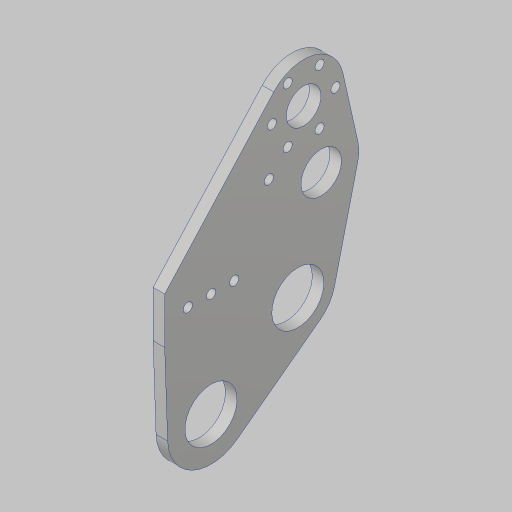
# Autodesk Inventor part: GP5-004
Saved by Autodesk Inventor 2023.5 (Build 275446000, 446)
## iProperties
Created: 2025-02-03
Part Number: GP5-004
Material: Aluminum 6061
Document SubType Name: Modeling
Designer: slick
Density: 2.7 g/cm^3
Appearance: Aluminum - Flat
Author: slick
Autodesk Inventor part; units mm, degrees
ref_plane "YZ Plane" through (0, 0, 0) normal (1, 0, 0) x (0, 1, 0)
ref_plane "XZ Plane" through (0, 0, 0) normal (0, 1, 0) x (-1, 0, 0)
ref_plane "XY Plane" through (0, 0, 0) normal (0, 0, 1) x (1, 0, 0)
sketch "Sketch1" plane through (0, 0, 0) normal (1, 0, 0) x (0, 1, 0)
  line L0 (-12.7, 25.4) -> (12.7, 25.4) construction
  line L1 (12.7, 25.4) -> (12.7, -25.4) construction
  line L2 (12.7, -25.4) -> (-12.7, -25.4) construction
  line L3 (-12.7, -25.4) -> (-12.7, 25.4) construction
  line L4 (-12.7, 25.4) -> (12.7, -25.4) construction
  line L5 (12.7, 25.4) -> (-12.7, -25.4) construction
  circle A0 centre (-57.15, 0) radius 14.2875
  circle A1 centre (-127, -49.5046) radius 38.1 construction
  circle A2 centre (-57.15, 0) radius 23.8125 construction
  circle A3 centre (63.9642, -50.8) radius 5.9531 construction
  circle A4 centre (27.5204, -60.4629) radius 31.75 construction
  circle A5 centre (63.9642, -50.8) radius 17.4625 construction
  circle A6 centre (63.9642, -50.8) radius 22.098 construction
  line L6 (12.7, -25.4) -> (215.9, -25.4) construction
  line L7 (215.9, -25.4) -> (215.9, 25.4) construction
  line L8 (215.9, 25.4) -> (12.7, 25.4) construction
  line L9 (-57.9919, 23.7976) -> (-12.7, 25.4)
  line L10 (-12.7, 25.4) -> (12.7, 25.4)
  line L11 (12.7, 25.4) -> (78.7925, -34.4157)
  arc A7 (68.7961, -72.3633) -> (78.7925, -34.4157) centre (63.9642, -50.8) ccw
  arc A8 (-57.9919, 23.7976) -> (-76.2318, -14.245) centre (-57.15, 0) ccw
  circle A9 centre (63.9642, -50.8) radius 9.525
  circle A10 centre (27.5204, -60.4629) radius 12.7 construction
  circle A11 centre (-25.5591, -47.625) radius 41.91 construction
  circle A12 centre (-25.5591, -47.625) radius 19.05 construction
  circle A13 centre (-57.15, 0) radius 38.1 construction
  circle A14 centre (27.5204, -60.4629) radius 11.1125
  circle A15 centre (-25.5591, -47.625) radius 14.2875
  circle A16 centre (27.5204, -60.4629) radius 20.6375 construction
  circle A17 centre (-25.5591, -47.625) radius 20.6375 construction
  line L12 (68.7961, -72.3633) -> (32.0329, -80.6011)
  line L13 (22.6689, -80.5221) -> (-30.4107, -67.6841)
  line L14 (-42.0967, -59.9706) -> (-76.2318, -14.245)
  arc A18 (22.6689, -80.5221) -> (32.0329, -80.6011) centre (27.5204, -60.4629) ccw
  arc A19 (-42.0967, -59.9706) -> (-30.4107, -67.6841) centre (-25.5591, -47.625) ccw
  circle A20 centre (38.5642, -31.75) radius 6.35 construction
  point P0 (0, 0)
  point P1 (0, -12.7)
  point P2 (0, 0)
  point P3 (0, 12.7)
  point P4 (-39.5444, 23.7687)
  point P5 (63.9642, -68.2625)
  point P6 (79.0872, -59.5312)
  point P7 (79.0872, -42.0688)
  point P8 (63.9642, -33.3375)
  point P9 (48.8413, -42.0687)
  point P10 (48.8413, -59.5312)
  dimension "d20" = 34.925
  dimension "d0" = 25.4
  dimension "d1" = 50.8
  dimension "d2" = 28.575
  dimension "d3" = 57.15
  dimension "d4" = 76.2
  dimension "d5" = 127
  dimension "d6" = 49.5046
  dimension "d11" = 12.7
  dimension "d12" = 12.7
  dimension "d13" = 9.525
  dimension "d18" = 11.9062
  dimension "d19" = 63.5
  dimension "d21" = 44.196
  dimension "d22" = 203.2
  dimension "d23" = 25.4
  dimension "d24" = 51.2642
  dimension "d27" = 19.05
  dimension "d31" = 360
  dimension "d40" = 25.4
  dimension "d41" = 83.82
  dimension "d42" = 38.1
  dimension "d43" = 76.2
  dimension "d44" = 36.4438
  dimension "d46" = 6.35
  dimension "d48" = 12.7
  dimension "d49" = 25.4
  dimension "d50" = 22.225
  dimension "d51" = 22.225
  constraints: 30 end point, 20 centre point, 16 point on circle, 13 coincident, 12 tangent, 5 vertical alignment, 3 equal radius, 3 perpendicular, 2 horizontal, 2 midpoint, 2 parallel, 1 horizontal alignment, 10 other
  measures "d0" distance of L1.end L2.end
  measures "d1" distance of L0.end L1.end
  measures "d2" diameter of A0
  measures "d3" distance of A0.centre point (0, 0)
  measures "d4" diameter of A1
  measures "d5" horizontal distance of A1.centre point (0, 0)
  measures "d6" vertical distance of A1.centre point (0, 0)
  measures "d11" distance of point (0, -12.7) point (0, 0)
  measures "d12" distance of point (0, 0) point (0, 12.7)
  measures "d13" radial gap between concentric circles of A0 A2
  measures "d18" diameter of A3
  measures "d19" diameter of A4
  measures "d21" diameter of A6
  measures "d22" distance between parallel lines of L1 L7
  measures "d23" distance from line of L6 point (63.964, -50.8)
  measures "d24" horizontal distance of L1.end A3.centre
  measures "d27" diameter of A9
  measures "d40" diameter of A10
  measures "d41" diameter of A11
  measures "d42" diameter of A12
  measures "d43" diameter of A13
  measures "d44" horizontal distance of A3.centre A4.centre
  measures "d46" radial gap between concentric circles of A15 A17
  measures "d48" diameter of A20
  measures "d49" horizontal distance of A20.centre A3.centre
  measures "d50" diameter of A14
  measures "d51" vertical distance of L2.end A11.centre
extrude "Extrusion1" add sketch "Sketch1" along normal blind 6.35
hole "Hole1" at (0, 0, -12.7) at (0, 0, 0) at (0, 0, 12.7) at (0, 63.9642, -68.2625) at (0, 79.0872, -59.5312) at (0, 79.0872, -42.0688) at (0, 63.9642, -33.3375) at (0, 48.8413, -42.0687) at (0, 48.8413, -59.5312) at (0, 38.5642, -31.75) direction (1, 0, 0) diameter 5.1054 end through all clearance for "Flat Head Machine Screw (82)" size "#10" standard "Ansi Unified Screw Threads"
equation "\"d12\" = d11"
body "Solid1"
